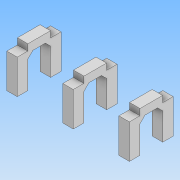
# Autodesk Inventor part: ViaductPillarsUnit
Saved by Autodesk Inventor 2021 (Build 250183000, 183)
## iProperties
Created: 2021-03-14
Part Number: ViaductPillarsUnit
Material: 一般
Document SubType Name: Modeling
Designer: kumagai
Density: 1 g/cm^3
Appearance: 既定
d0: 117.500 mm
d2: 10.000 mm
d3: 10.000 mm
d4: 33.000 mm
d5: 0.00 deg
d10: 3.000 mm
d11: 3.000 mm
d13: 3.000 mm
d14: 6.000 mm
d15: 0.00 deg
d25: 8.000 mm
d26: 0.00 deg
d27: 6.000 mm
d28: 0.00 deg
d35: 0.150 mm
d37: 39.000 mm
d92: 3.000 mm
d94: 5.000 mm
d99: 45.00 deg
d100: 45.00 deg
d101: 3.000 mm
d104: 1.000 mm
UnitHeight: 33.000 mm
ID: 3.000 mm
VPW: 10.000 mm
VBW: 8.000 mm
OF: 0.150 mm
PrinterOffset: 0.000 mm
StraightLength: 215.000 mm
RailWidth: 38.000 mm
OuterWall: 2.000 mm
InnerWall: 2.400 mm
InsideWidth: 18.600 mm
RailHeight: 8.400 mm
RailDepth: 3.200 mm
ConnectorLength: 15.000 mm
ViaductHeight: 66.000 mm
Author: kumagai
Autodesk Inventor part; units mm, degrees
ref_plane "YZ Plane" through (0, 0, 0) normal (1, 0, 0) x (0, 1, 0)
ref_plane "XY Plane" through (0, 0, 0) normal (0, 0, 1) x (1, 0, 0)
sketch "スケッチ1" plane through (0, 0, 0) normal (0, 1, 0) x (-1, 0, 0)
  line L0 (-58.75, -21) -> (-58.75, 21)
  line L1 (58.75, 21) -> (58.75, -21)
  line L2 (0, -29.4) -> (0, 29.4) projected
  line L3 (-82.25, 0) -> (82.25, 0) projected
  line L4 (58.75, -21) -> (48.75, -21)
  line L5 (48.75, -21) -> (48.75, -11)
  line L6 (48.75, -11) -> (58.75, -11)
  line L7 (58.75, -11) -> (58.75, -21)
  line L8 (5, -21) -> (-5, -21)
  line L9 (-5, -21) -> (-5, -11)
  line L10 (-5, -11) -> (5, -11)
  line L11 (5, -11) -> (5, -21)
  line L12 (-48.75, -21) -> (-58.75, -21)
  line L13 (-58.75, -21) -> (-58.75, -11)
  line L14 (-58.75, -11) -> (-48.75, -11)
  line L15 (-48.75, -11) -> (-48.75, -21)
  line L16 (-58.75, 11) -> (-48.75, 11)
  line L17 (-48.75, 11) -> (-48.75, 21)
  line L18 (-48.75, 21) -> (-58.75, 21)
  line L19 (-58.75, 21) -> (-58.75, 11)
  line L20 (5, 21) -> (-5, 21)
  line L21 (-5, 21) -> (-5, 11)
  line L22 (-5, 11) -> (5, 11)
  line L23 (5, 11) -> (5, 21)
  line L24 (58.75, 11) -> (48.75, 11)
  line L25 (48.75, 11) -> (48.75, 21)
  line L26 (48.75, 21) -> (58.75, 21)
  line L27 (58.75, 21) -> (58.75, 11)
  line L28 (5, -11) -> (5, 11)
  line L29 (48.75, 11) -> (48.75, -11)
  line L30 (-48.75, -11) -> (-48.75, 11)
  line L31 (-5, 11) -> (-5, -11)
  line L32 (55.75, 11) -> (55.75, -11)
  line L33 (-55.75, -11) -> (-55.75, 11)
  line L34 (2, 11) -> (2, -11)
  line L35 (-2, -11) -> (-2, 11)
  line L36 (51.75, -11) -> (51.75, 11)
  line L37 (-51.75, -11) -> (-51.75, 11)
  line L38 (-58.75, 21) -> (-48.75, 21)
  line L39 (-5, 21) -> (5, 21)
  line L40 (48.75, 21) -> (58.75, 21)
  line L41 (58.75, -21) -> (48.75, -21)
  line L42 (5, -21) -> (-5, -21)
  line L43 (-48.75, -21) -> (-58.75, -21)
  point P0 (0, 0)
  dimension "d0" = 117.5
  dimension "d2" = 10
  dimension "d10" = 3
  dimension "d13" = 3
  dimension "d92" = 3
  dimension "d119" = 22
  dimension "d120" = 10
  constraints: 84 end point, 25 parallel, 16 point on line, 11 collinear, 11 perpendicular, 9 horizontal, 1 vertical, 10 other
  measures "d0" distance between parallel lines of L0 L1
  measures "d2" distance between parallel lines of L21 L23
  measures "d10" distance between parallel lines of L1 L32
  measures "d13" distance between parallel lines of L28 L34
  measures "d92" distance between parallel lines of L29 L36
  measures "d119" distance between parallel lines of L14 L16
  measures "d120" distance between parallel lines of L16 L18
extrude "押し出し1" add sketch "スケッチ1" along normal blind 33 contours L0 L14 L15 L12 | L0 L18 L17 L16 | L1 L24 L25 L26 | L1 L4 L5 L6 | L8 L9 L10 L2 | L2 L10 L11 L8 | L22 L21 L20 L2 | L2 L20 L23 L22
extrude "押し出し4" [suppressed]
ref_plane "作業平面2" through (0, 39, 0) normal (0, 1, 0) x (-1, 0, 0)
sketch "スケッチ2" plane through (0, 39, 0) normal (0, 1, 0) x (-1, 0, 0)
  line L0 (58.75, 21) -> (58.75, -21) projected
  line L1 (55.75, 11) -> (55.75, -11) projected
  line L2 (51.75, -11) -> (51.75, 11) projected
  line L3 (48.75, 11) -> (48.75, -11) projected
  line L4 (58.75, 11) -> (48.75, 11) projected
  line L5 (48.75, -11) -> (58.75, -11) projected
  line L6 (58.75, -21) -> (48.75, -21) projected
  line L7 (48.75, -21) -> (48.75, -11) projected
  line L8 (48.75, 11) -> (48.75, 21) projected
  line L9 (5, 11) -> (5, 21) projected
  line L10 (-5, 11) -> (5, 11) projected
  line L11 (-5, 21) -> (-5, 11) projected
  line L12 (5, -11) -> (5, -21) projected
  line L13 (-5, -11) -> (5, -11) projected
  line L14 (-5, -21) -> (-5, -11) projected
  line L15 (5, -21) -> (-5, -21) projected
  line L16 (-5, 11) -> (-5, -11) projected
  line L17 (-2, -11) -> (-2, 11) projected
  line L18 (2, 11) -> (2, -11) projected
  line L19 (5, -11) -> (5, 11) projected
  line L20 (-48.75, 11) -> (-48.75, 21) projected
  line L21 (-48.75, -11) -> (-48.75, 11) projected
  line L22 (-48.75, -11) -> (-48.75, -21) projected
  line L23 (-58.75, -21) -> (-58.75, 21) projected
  line L24 (-58.75, -11) -> (-48.75, -11) projected
  line L25 (-58.75, 11) -> (-48.75, 11) projected
  line L26 (-51.75, -11) -> (-51.75, 11) projected
  line L27 (-55.75, -11) -> (-55.75, 11) projected
extrude "押し出し6" add sketch "スケッチ2" against normal blind 8 contours L0 L5 L1 L4 | L1 L5 L2 L4 | L2 L5 L3 L4 | L10 L17 L13 L16 | L10 L18 L13 L17 | L10 L19 L13 L18 | L24 L26 L25 L21 | L24 L27 L25 L26 | L24 L23 L25 L27
extrude "押し出し7" [suppressed]
thicken "厚み1" operation cut thickness 0.15 both sides no extend neighbours no toward (0, -1, 0) faces at (55.4167, 33, -14.3333) (55.4167, 33, 17.6667) (52.0833, 37, 11) (55.4167, 37, -11) (55.4167, 39, 3.6667)
thicken "厚み2" operation cut thickness 0.15 both sides no extend neighbours no toward (0, -1, 0) faces at (1.6667, 33, -14.3333) (1.6667, 33, 17.6667) (1.6667, 39, 3.6667) (1.6667, 37, -11) (-1.6667, 37, 11)
thicken "厚み3" operation cut thickness 0.15 both sides no extend neighbours no toward (0, -1, 0) faces at (-52.0833, 33, -14.3333) (-52.0833, 33, 17.6667) (-55.4167, 37, 11) (-55.4167, 39, -3.6667) (-52.0833, 37, -11)
sketch "SupportBase" plane through (0, 0, 0) normal (0, -1, 0) x (1, 0, 0)
  line L0 (-48.75, 11) -> (-48.75, -11)
  line L1 (-48.75, -11) -> (-5, -11)
  line L2 (-48.75, 11) -> (-5, 11)
  line L3 (-5, 11) -> (-5, -11)
  line L4 (5, 11) -> (5, -11)
  line L5 (5, -11) -> (48.75, -11)
  line L6 (48.75, -11) -> (48.75, 11)
  line L7 (5, 11) -> (48.75, 11)
  constraints: 16 end point
sketch "SupportTarget" plane through (0, 31, 0) normal (0, -1, 0) x (1, 0, 0)
  line L0 (48.75, 11) -> (58.75, 11) projected
  line L1 (48.75, 11) -> (48.75, -11) projected
  line L2 (58.75, -11) -> (48.75, -11) projected
  line L3 (58.75, -11) -> (58.75, 11) projected
  line L4 (-5, 11) -> (5, 11) projected
  line L5 (-5, 11) -> (-5, -11) projected
  line L6 (5, -11) -> (-5, -11) projected
  line L7 (5, -11) -> (5, 11) projected
  line L8 (-58.75, 11) -> (-58.75, -11) projected
  line L9 (-48.75, -11) -> (-58.75, -11) projected
  line L10 (-48.75, -11) -> (-48.75, 11) projected
  line L11 (-58.75, 11) -> (-48.75, 11) projected
chamfer "面取り6" distance 5 angle 45 6 edges at (-53.75, 31, -11) (0, 31, -11) (53.75, 31, -11) (-53.75, 31, 11) (0, 31, 11) (53.75, 31, 11)
equation "\"d2\" = VPW"
equation "\"d10\" = ID"
equation "\"d13\" = ID"
equation "\"d4\" = UnitHeight"
equation "\"d14\" = 2 * ID"
equation "\"d25\" = VBW"
equation "\"d27\" = 2 * ID"
equation "\"d36\" = OF"
equation "\"d3\" = VPW"
equation "\"UnitHeight\" = 0.5 * ViaductHeight"
equation "\"ID\" = 3"
equation "\"VPW\" = 10"
equation "\"d11\" = ID"
equation "\"VBW\" = 8"
equation "\"OF\" = 0.15"
equation "\"d37\" = UnitHeight + 2 * ID"
equation "\"ViaductHeight\" = 66"
